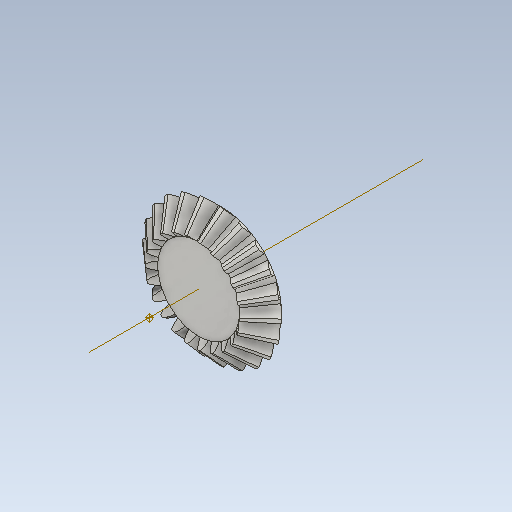
# Autodesk Inventor part: Kegelrad1
Saved by Autodesk Inventor 2021 (Build 250183000, 183)
## iProperties
CustomPartVersion: 1
Created: 2021-01-22
Part Number: Kegelrad1
Material: Steel, Mild
Document SubType Name: Modeling
Designer: Jaro Machnow
Categories: <?xml version="1.0" encoding="UTF-16"?> <MemberInstance><Categories><FamilyTemplate><FamilyTemplateParameter ValueType="xs:double" Id="1" ObjectReferenceKey="da_z" ObjectType="kUserParameterObject"/><FamilyTemplateParameter ValueType="xs:double" Id="2" ObjectReferenceKey="da_b" ObjectType="kUserParameterObject"/><FamilyTemplateParameter ValueType="xs:double" Id="3" ObjectReferenceKey="da_beta" ObjectType="kUserParameterObject"/><FamilyTemplateParameter ValueType="xs:double" Id="4" ObjectReferenceKey="da_dae" ObjectType="kUserParameterObject"/><FamilyTemplateParameter ValueType="xs:double" Id="5" ObjectReferenceKey="da_ve" ObjectType="kUserParameterObject"/><FamilyTemplateParameter ValueType="xs:double" Id="6" ObjectReferenceKey="da_omega" ObjectType="kUserParameterObject"/><FamilyTemplateParameter ValueType="xs:string" Id="7" ObjectReferenceKey="EAIAABAAAAAAHwAAAAAAAIAAAAAAAAAA" ObjectType="83914240" SubObjectId="SurfaceGeometry"/></FamilyTemplate><ParamToTemplateMap><ParamToTemplate CategoryParameter="//CategoryParameter[@InternalName='046C89C9-8512-4d59-83FE-43B91F4F132A']" TemplateParameter="1"/><ParamToTemplate CategoryParameter="//CategoryParameter[@InternalName='2552DF32-E462-4b46-AEBF-C6C7768E72AC']" TemplateParameter="2"/><ParamToTemplate CategoryParameter="//CategoryParameter[@InternalName='C9EE641D-15FC-4fae-A226-E94C4372FDD7']" TemplateParameter="3"/><ParamToTemplate><ParamToTemplate CategoryParameter="//CategoryParameter[@InternalName='00B6519A-459B-49c7-AD84-2E56D39A5744']" ConstantValue="0.000000"/></ParamToTemplate><ParamToTemplate><ParamToTemplate CategoryParameter="//CategoryParameter[@InternalName='04B31F0E-C7A6-4894-AA32-9629BEFACF47']" ConstantValue="1.000000"/></ParamToTemplate><ParamToTemplate><ParamToTemplate CategoryParameter="//CategoryParameter[@InternalName='43CBEC2E-7847-49e7-A936-2F7889FCB2D9']" ConstantValue="0.200000"/></ParamToTemplate><ParamToTemplate><ParamToTemplate CategoryParameter="//CategoryParameter[@InternalName='B1EFC894-105D-4ebd-86BF-FA20ED196853']" ConstantValue="0.300000"/></ParamToTemplate><ParamToTemplate><ParamToTemplate CategoryParameter="//CategoryParameter[@InternalName='51175063-3D10-4879-93E8-6246FE8B403D']" ConstantValue="2060000000.000000"/></ParamToTemplate><ParamToTemplate><ParamToTemplate CategoryParameter="//CategoryParameter[@InternalName='A3A52E27-4454-46a9-B0BD-C932399B70AF']" ConstantValue="0.300000"/></ParamToTemplate><ParamToTemplate CategoryParameter="//CategoryParameter[@InternalName='2A200944-5A8C-41ca-B96E-8520D2E510F1']" TemplateParameter="4"/><ParamToTemplate><ParamToTemplate CategoryParameter="//CategoryParameter[@InternalName='1A637F62-92C8-44bc-B81F-10802510B579']" ConstantValue="1.112202"/></ParamToTemplate><ParamToTemplate CategoryParameter="//CategoryParameter[@InternalName='B52DD4BE-6863-48fb-BF58-89EF6F9EC65C']" TemplateParameter="5"/><ParamToTemplate><ParamToTemplate CategoryParameter="//CategoryParameter[@InternalName='3956BFF2-84D2-457d-93C2-9B0613DEBA67']" ConstantValue="0.488924"/></ParamToTemplate><ParamToTemplate CategoryParameter="//CategoryParameter[@InternalName='739CFA02-461B-4bf8-8049-181FCAD8B28F']" TemplateParameter="6"/><ParamToTemplate><ParamToTemplate CategoryParameter="//CategoryParameter[@InternalName='A27E999F-E2CE-4481-8A2A-EBF499C4C3C5']" ConstantValue="0.000000"/></ParamToTemplate><ParamToTemplate><ParamToTemplate CategoryParameter="//CategoryParameter[@InternalName='9E1B4470-B2D3-4ff1-B813-535BB4CDF51A']" ConstantValue="3520000.000000"/></ParamToTemplate><ParamToTemplate><ParamToTemplate CategoryParameter="//CategoryParameter[@InternalName='F8452263-BFF6-458c-9FB1-07C4B99E95CD']" ConstantValue="11400000.000000"/></ParamToTemplate><ParamToTemplate><ParamToTemplate CategoryParameter="//CategoryParameter[@InternalName='3E3BB259-FD49-497f-8171-6EBC954A3479']" ConstantValue="2.000000"/></ParamToTemplate><ParamToTemplate CategoryParameter="//CategoryParameter[@InternalName='27C3BAF2-7550-4e4b-AE2C-0DB134B7D9B7']" TemplateParameter="7"/></ParamToTemplateMap><Category DisplayName="Gear" InternalName="DC85795E-93AB-48d5-8EEE-5A27447B64BD" Mnemonic="Gear"><CategoryParameter DisplayName="z" InternalName="046C89C9-8512-4d59-83FE-43B91F4F132A" Mnemonic="z"/><CategoryParameter DisplayName="b" InternalName="2552DF32-E462-4b46-AEBF-C6C7768E72AC" Mnemonic="b"/><CategoryParameter DisplayName="||b|" InternalName="C9EE641D-15FC-4fae-A226-E94C4372FDD7" Mnemonic="beta"/><CategoryParameter DisplayName="x" InternalName="00B6519A-459B-49c7-AD84-2E56D39A5744" Mnemonic="x"/><CategoryParameter DisplayName="a*" InternalName="04B31F0E-C7A6-4894-AA32-9629BEFACF47" Mnemonic="a"/><CategoryParameter DisplayName="c*" InternalName="43CBEC2E-7847-49e7-A936-2F7889FCB2D9" Mnemonic="c"/><CategoryParameter DisplayName="r|.f|*" InternalName="B1EFC894-105D-4ebd-86BF-FA20ED196853" Mnemonic="rf"/><CategoryParameter DisplayName="E" InternalName="51175063-3D10-4879-93E8-6246FE8B403D" Mnemonic="E"/><CategoryParameter DisplayName="||m|" InternalName="A3A52E27-4454-46a9-B0BD-C932399B70AF" Mnemonic="mi"/><Category DisplayName="BevelGear" InternalName="0C98F69A-0C2B-4791-B2FE-7691BB227E77" Mnemonic="BevelGear"><CategoryParameter DisplayName="d|.ae|" InternalName="2A200944-5A8C-41ca-B96E-8520D2E510F1" Mnemonic="dae"/><CategoryParameter DisplayName="d|.ai|" InternalName="1A637F62-92C8-44bc-B81F-10802510B579" Mnemonic="dai"/><CategoryParameter DisplayName="A|.e|" InternalName="B52DD4BE-6863-48fb-BF58-89EF6F9EC65C" Mnemonic="ve"/><CategoryParameter DisplayName="A|.i|" InternalName="3956BFF2-84D2-457d-93C2-9B0613DEBA67" Mnemonic="vi"/><CategoryParameter DisplayName="||S|" InternalName="739CFA02-461B-4bf8-8049-181FCAD8B28F" Mnemonic="omega"/><CategoryParameter DisplayName="x|.t|" InternalName="A27E999F-E2CE-4481-8A2A-EBF499C4C3C5" Mnemonic="xt"/><CategoryParameter DisplayName="||s||.Flim|" InternalName="9E1B4470-B2D3-4ff1-B813-535BB4CDF51A" Mnemonic="sFlim"/><CategoryParameter DisplayName="||s||.Hlim|" InternalName="F8452263-BFF6-458c-9FB1-07C4B99E95CD" Mnemonic="sHlim"/><CategoryParameter DisplayName="Typ" InternalName="3E3BB259-FD49-497f-8171-6EBC954A3479" Mnemonic="type"/><CategoryParameter DisplayName="PitchDiameter" InternalName="27C3BAF2-7550-4e4b-AE2C-0DB134B7D9B7" Mnemonic="IDS_PITCHDIAM"/></Category></Category></Categories></MemberInstance>
Mass: 60.9118 g
Surface Area: 34.3074 cm^2
Volume: 7.7496 cm^3
Density: 7.86 g/cm^3
Appearance: Steel
Author: Jaro Machnow
Autodesk Inventor part; units mm, degrees
ref_plane "Netzebene2" through (0, 0, 0) normal (0.9898214, 0.1423148, 0) x (0, 0, 1)
sketch "Skizze des Zahnradkörpers" plane through (0, 0, 0) normal (1, 0, 0) x (0, 1, 0)
  line L0 (0, 0) -> (7.106, -8.294) construction
  line L1 (7.106, -8.294) -> (8.195, -7.205)
  line L2 (8.195, -7.205) -> (0, 0) construction
  line L3 (7.7, -7.7) -> (0, 0) construction
  line L4 (4.8221, -5.6282) -> (5.561, -4.8892)
  line L5 (7.106, -8.294) -> (4.8221, -5.6282)
  line L6 (8.195, -7.205) -> (5.561, -4.8892)
  line L7 (0, -10.3728) -> (0, 1.7288) projected
  line L8 (0, -7.7) -> (8.195, -7.7) construction
  dimension "d0" = 15.4
  dimension "d1" = 14.2121
  dimension "d2" = 16.3899
  dimension "d3" = 3.5
  dimension "d4" = 7.205
  constraints: 16 end point, 4 point on line, 3 perpendicular, 2 collinear, 1 horizontal alignment, 1 vertical alignment
  measures "d0" diameter of L3.start L7
  measures "d1" diameter of L0.end L7
  measures "d2" diameter of L1.end L7
  measures "d3" distance between parallel lines of L1 L4
  measures "d4" vertical distance of L1.end L0.start
revolve "Zahnradkörper" add sketch "Skizze des Zahnradkörpers" angle 360 about axis through (0, 0, 0) along (0, 0, 1)
ref_plane "Zahnebene" through (0, 7.7, -7.7) normal (0, -0.7071068, 0.7071068) x (1, 0, 0)
sketch "Startskizze" plane through (0, 7.7, -7.7) normal (0, -0.7071068, 0.7071068) x (1, 0, 0)
  line L0 (0, -13.8953) -> (0, 3.681) projected
  arc A0 (-0.2755, -1.0248) -> (-1.267, 1.0952) centre (-4.2013, -1.5689) ccw
  arc A1 (1.267, 1.0952) -> (0.2755, -1.0248) centre (4.2013, -1.5689) ccw
  line L1 (-0.2755, -1.0248) -> (0.2755, -1.0248)
  arc A2 (1.267, 1.0952) -> (-1.267, 1.0952) centre (0, -10.8894) ccw
  dimension "d7" = 3.9633
  dimension "d8" = 4.2012
  dimension "d9" = 9.3205
  dimension "d57" = 12.0514
  dimension "d58" = 9.8646
  constraints: 6 point on circle, 3 centre point, 3 symmetric about line, 2 end point, 1 coincident, 1 perpendicular, 1 other
  measures "d7" radius of A0
  measures "d8" horizontal distance of point (0, -10.889) A0.centre
  measures "d9" vertical distance of point (0, -10.889) A0.centre
  measures "d57" radius of A2
  measures "d58" distance from line of A2.centre L1
ref_plane "Endebene" through (0, 5.1707, -5.1707) normal (0, -0.7071068, 0.7071068) x (1, 0, 0)
sketch "Endskizze" plane through (0, 5.1707, -5.1707) normal (0, -0.7071068, 0.7071068) x (1, 0, 0)
  line L0 (0, -9.5294) -> (0, 2.5244) projected
  arc A0 (-0.185, -0.6882) -> (-0.8508, 0.7355) centre (-2.8212, -1.0536) ccw
  arc A1 (0.8508, 0.7355) -> (0.185, -0.6882) centre (2.8212, -1.0536) ccw
  line L1 (-0.185, -0.6882) -> (0.185, -0.6882)
  arc A2 (0.8508, 0.7355) -> (-0.8508, 0.7355) centre (0, -7.3124) ccw
  dimension "d12" = 2.6614
  dimension "d15" = 2.8212
  dimension "d16" = 6.2589
  dimension "d59" = 8.0928
  dimension "d60" = 6.6243
  constraints: 6 point on circle, 3 centre point, 3 symmetric about line, 2 end point, 1 coincident, 1 other
  measures "d12" radius of A0
  measures "d15" horizontal distance of A0.centre point (0, -7.312)
  measures "d16" vertical distance of A0.centre point (0, -7.312)
  measures "d59" radius of A2
  measures "d60" distance from line of A2.centre L1
loft "Loft" cut profiles "Startskizze", "Endskizze"
pattern_circular "Circular Pattern" count 22 over 360 about axis through (0, 0, 0) along (0, 0, 1) of "Loft"
sketch3d "3D-Skizze rechts"
ref_plane "Endebene rechts" through (-0.9538, 5.082, -5.1707) normal (0.1304331, -0.6949728, 0.7071068) x (0.98284, 0.1844602, 0)
sketch "Endskizze rechts" plane through (-0.9538, 5.082, -5.1707) normal (0.1304331, -0.6949728, 0.7071068) x (0.98284, 0.1844602, 0)
  arc A0 (-0.185, -0.6882) -> (-0.8508, 0.7355) centre (-2.8212, -1.0536) ccw
  line L0 (0, -10.6032) -> (0, 3.5982) projected
  arc A1 (0.8508, 0.7355) -> (0.185, -0.6882) centre (2.8212, -1.0536) ccw
  line L1 (-0.185, -0.6882) -> (0.185, -0.6882)
  arc A2 (0.8508, 0.7355) -> (-0.8508, 0.7355) centre (0, -7.3124) ccw
  dimension "d70" = 2.8212
  dimension "d71" = 6.2589
  dimension "d72" = 2.6614
  dimension "d73" = 6.6243
  dimension "d74" = 8.0928
  constraints: 6 point on circle, 3 centre point, 3 symmetric about line, 2 end point, 1 coincident, 1 perpendicular, 1 other
  measures "d70" horizontal distance of A2.centre A0.centre
  measures "d71" vertical distance of point (0, -7.312) A0.centre
  measures "d72" radius of A0
  measures "d73" distance from line of point (0, -7.312) L1
  measures "d74" radius of A2
feature "Erhebung rechts" [suppressed]
pattern_circular "Runde Anordnung rechts" [suppressed]
sketch3d "3D-Skizze links"
ref_plane "Endebene links" through (0.9889, 5.082, -5.1842) normal (-0.1349695, -0.6936245, 0.7075792) x (0.9815894, -0.1910033, 0)
sketch "Endskizze links" plane through (0.9889, 5.082, -5.1842) normal (-0.1349695, -0.6936245, 0.7075792) x (0.9815894, -0.1910033, 0)
  line L0 (0, -11.8215) -> (0, 4.7448) projected
  arc A0 (-0.185, -0.6833) -> (-0.8508, 0.7403) centre (-2.8212, -1.0487) ccw
  arc A1 (0.8508, 0.7403) -> (0.185, -0.6833) centre (2.8212, -1.0487) ccw
  line L1 (-0.185, -0.6833) -> (0.185, -0.6833)
  ellipse E0 centre (0, -3.4549) end of major axis (5.561, -3.4549) minor radius 3.9349 projected
  arc A2 (0.8508, 0.7403) -> (-0.8508, 0.7403) centre (0, -7.3076) ccw
  dimension "d56" = 3.9348
  dimension "d30" = 2.6614
  dimension "d31" = 2.8212
  dimension "d32" = 6.2589
  dimension "d61" = 8.0928
  dimension "d62" = 6.6243
  constraints: 6 point on circle, 3 centre point, 3 symmetric about line, 2 end point, 1 coincident, 2 other
  measures "d30" radius of A0
  measures "d31" horizontal distance of point (0, -7.308) A0.centre
  measures "d32" vertical distance of A0.centre point (0, -7.308)
  measures "d61" radius of A2
  measures "d62" distance from line of point (0, -7.308) L1
feature "Erhebung links" [suppressed]
pattern_circular "Runde Anordnung links" [suppressed]
sketch "Körperskizze" plane through (0, 0, 0) normal (1, 0, 0) x (0, 1, 0)
  line L0 (0, -9.1755) -> (0, -5.455) projected
  line L1 (7.106, -8.294) -> (4.8221, -5.6282) projected
  line L2 (4.8221, -5.6282) -> (0, -5.6282)
  line L3 (7.106, -8.294) -> (0, -8.294)
  constraints: 4 end point, 2 perpendicular, 2 point on line
revolve "Festkörper" add sketch "Körperskizze" angle 360 about axis through (0, 0, 0) along (0, 0, 1)
sketch "Sketch6" plane through (0, 0, 0) normal (1, 0, 0) x (0, 1, 0)
  line L0 (7.7, -7.7) -> (0, 0) projected
  line L1 (0, -9.66) -> (0, 1.61) projected
surface revolve "Flankendurchmesser" sketch "Sketch6" angle 360 about axis through (0, 0, 0) along (0, 0, 1) shown no curves L0
equation "\"d0\" = da_de"
equation "\"d1\" = da_dfe"
equation "\"d2\" = da_dae"
equation "\"d3\" = da_b"
equation "\"d4\" = da_ve"
equation "\"d7\" = fd_rr"
equation "\"d8\" = fd_x"
equation "\"d9\" = fd_y"
equation "\"d57\" = 0.5 * fd_dva + 0.3 * da_he"
equation "\"d58\" = 0.5 * fd_dva - 1.12 * da_he"
equation "\"da_teethtype\" = 0"
equation "\"da_b\" = 3.5"
equation "\"da_de\" = 15.4"
equation "\"da_dae\" = 16.38995"
equation "\"da_dfe\" = 14.21206"
equation "\"da_le\" = 10.88944"
equation "\"da_omega\" = 90deg"
equation "\"da_beta\" = 0"
equation "\"da_delta\" = 45deg"
equation "\"da_alpha\" = 20deg"
equation "\"da_he\" = 1.54"
equation "\"da_ve\" = 7.20503"
equation "\"da_zv\" = 31.112698"
equation "\"fd_loft\" = da_b + 0.05 * da_he"
equation "\"fd_x\" = fd_x1 + fd_x2"
equation "\"fd_y\" = fd_y1 - fd_y2"
equation "\"fd_dd\" = fd_dva - 0.8 * da_he"
equation "\"da_dvw\" = 21.77889"
equation "\"d11\" = fd_loft"
equation "\"da_dm\" = 12.92513"
equation "\"da_x\" = 0"
equation "\"da_m\" = 0.7"
equation "\"d50\" = da_omega"
equation "\"fd_rr\" = 3.963295"
equation "\"fd_dva\" = 23.178889"
equation "\"fd_x1\" = 0.555646"
equation "\"fd_x2\" = 3.645605"
equation "\"fd_y1\" = 10.875259"
equation "\"fd_y2\" = 1.554757"
body "Solid1"
body "Srf1"
